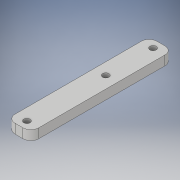
# Autodesk Inventor part: ArmLifter
Saved by Autodesk Inventor 2019 (Build 230136000, 136)
## iProperties
Created: 2018-06-10
Part Number: ArmLifter
Material: Ogólny
Document SubType Name: Modeling
Designer: Kamil
Density: 1 g/cm^3
Appearance: Domyślna
Author: Kamil
Autodesk Inventor part; units mm, degrees
ref_plane "YZ Plane" through (0, 0, 0) normal (1, 0, 0) x (0, 1, 0)
ref_plane "XZ Plane" through (0, 0, 0) normal (0, 1, 0) x (-1, 0, 0)
ref_plane "XY Plane" through (0, 0, 0) normal (0, 0, 1) x (1, 0, 0)
sketch "Szkic1" plane through (0, 0, 0) normal (0, 1, 0) x (-1, 0, 0)
  line L0 (2.5, -45) -> (-2.5, -45)
  line L1 (-7.5, -40) -> (-7.5, 40)
  line L2 (-2.5, 45) -> (2.5, 45)
  line L3 (7.5, 40) -> (7.5, -40)
  line L4 (7.5, -45) -> (-7.5, 45) construction
  line L5 (-7.5, -45) -> (7.5, 45) construction
  arc A0 (7.5, 40) -> (2.5, 45) centre (2.5, 40) ccw
  arc A1 (-2.5, 45) -> (-7.5, 40) centre (-2.5, 40) ccw
  arc A2 (2.5, -45) -> (7.5, -40) centre (2.5, -40) ccw
  arc A3 (-7.5, -40) -> (-2.5, -45) centre (-2.5, -40) ccw
  circle A4 centre (0, 40) radius 2
  circle A5 centre (0, -10) radius 2
  circle A6 centre (0, -40) radius 2
  point P0 (0, 0)
  dimension "d0" = 15
  dimension "d1" = 90
  dimension "d2" = 5
  dimension "d3" = 4
  dimension "d4" = 4
  dimension "d5" = 4
  constraints: 12 end point, 8 point on circle, 8 point on line, 8 tangent, 7 centre point, 3 equal radius, 2 midpoint, 2 parallel, 1 horizontal, 1 perpendicular
  measures "d0" distance of L4.end L5.end
  measures "d1" distance of L5.start L4.end
  measures "d2" radius of A0
  measures "d3" diameter of A4
  measures "d4" diameter of A5
  measures "d5" diameter of A6
extrude "Wyciągnięcie proste1" add sketch "Szkic1" along normal blind 6
